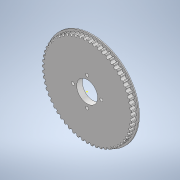
# Autodesk Inventor part: プーリ_歯数60_関節1
Saved by Autodesk Inventor 2021 (Build 250183000, 183)
## iProperties
Created: 2022-02-01
Part Number: プーリ_歯数60_関節1
Material: 一般
Document SubType Name: Modeling
Designer: hirohumi
Density: 1 g/cm^3
Appearance: 既定
Author: hirohumi
Autodesk Inventor part; units mm, degrees
ref_plane "YZ Plane" through (0, 0, 0) normal (1, 0, 0) x (0, 1, 0)
ref_plane "XZ Plane" through (0, 0, 0) normal (0, 1, 0) x (-1, 0, 0)
ref_plane "XY Plane" through (0, 0, 0) normal (0, 0, 1) x (1, 0, 0)
sketch "スケッチ1" plane through (0, 0, 0) normal (0, 0, 1) x (1, 0, 0)
  arc A0 (11.2031, 43.8361) -> (-12.7392, 43.4146) centre (0, 0) ccw construction
  arc A1 (-0.569, 47.1716) -> (-1.072, 46.6316) centre (-0.5629, 46.6616) ccw
  arc A2 (1.072, 46.6316) -> (0.569, 47.1716) centre (0.5629, 46.6616) ccw
  arc A3 (-2.3679, 45.183) -> (-1.072, 46.6316) centre (-2.4396, 46.5511) ccw
  arc A4 (1.072, 46.6316) -> (2.3679, 45.183) centre (2.4396, 46.5511) ccw
  arc A5 (0.569, 47.1716) -> (-0.569, 47.1716) centre (0, 0) ccw
  line L0 (-2.3679, 45.183) -> (0, 0)
  line L1 (0, 0) -> (2.3679, 45.183)
  line L2 (0, 0) -> (0, 8.5337) construction
  dimension "d4" = 0.51
  dimension "d5" = 0.51
  dimension "d6" = 1.37
  dimension "d7" = 1.37
  dimension "d8" = 6
  dimension "d9" = 3
  dimension "d20" = 47.175
  dimension "d21" = 1.93
  constraints: 14 point on circle, 6 centre point, 6 end point, 6 tangent, 2 coincident, 1 vertical
  measures "d4" radius of A1
  measures "d5" radius of A2
  measures "d6" radius of A3
  measures "d7" radius of A4
  measures "d8" angle of L1 L0
  measures "d9" angle of L2 L0
  measures "d20" radius of A5
  measures "d21" radial gap between concentric circles of A0 A5
extrude "押し出し1" add sketch "スケッチ1" along normal blind 5
pattern_circular "円形状パターン1" count 60 over 360 about axis through (0, 0, 0) along (0, 0, 1) of "押し出し1"
sketch "スケッチ2" plane through (0, 0, 0) normal (0, 0, -1) x (-1, 0, 0)
  circle A0 centre (0, 0) radius 49
  dimension "d15" = 98
  constraints: 1 centre point, 1 coincident
  measures "d15" diameter of A0
extrude "押し出し2" add sketch "スケッチ2" along normal blind 1
sketch "スケッチ3" plane through (0, 0, 5) normal (0, 0, 1) x (1, 0, 0)
  point P0 (0, 0)
sketch "スケッチ4" plane through (0, 0, 5) normal (0, 0, 1) x (1, 0, 0)
  circle A0 centre (0, 0) radius 11.05
  circle A1 centre (0, 15) radius 1.6
  circle A2 centre (-15, 0) radius 1.6
  circle A3 centre (0, -15) radius 1.6
  circle A4 centre (15, 0) radius 1.6
  circle A5 centre (0, 0) radius 15 construction
  dimension "d23" = 22.1
  dimension "d24" = 3.2
  dimension "d25" = 3.2
  dimension "d26" = 3.2
  dimension "d27" = 3.2
  dimension "d28" = 30
  constraints: 6 centre point, 4 point on circle, 2 coincident, 2 horizontal alignment, 2 vertical alignment
  measures "d23" diameter of A0
  measures "d24" diameter of A1
  measures "d25" diameter of A2
  measures "d26" diameter of A3
  measures "d27" diameter of A4
  measures "d28" diameter of A5
extrude "押し出し3" cut sketch "スケッチ4" against normal through all
